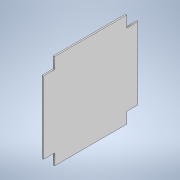
# Autodesk Inventor part: Frame
Saved by Autodesk Inventor 2022 (Build 260153000, 153)
## iProperties
Created: 2022-02-12
Part Number: Frame
Material: Generic
Document SubType Name: Modeling
Designer: ultra
Density: 1 g/cm^3
Appearance: Default
Author: ultra
Autodesk Inventor part; units mm, degrees
ref_plane "YZ Plane" through (0, 0, 0) normal (1, 0, 0) x (0, 1, 0)
ref_plane "XZ Plane" through (0, 0, 0) normal (0, 1, 0) x (-1, 0, 0)
ref_plane "XY Plane" through (0, 0, 0) normal (0, 0, 1) x (1, 0, 0)
sketch "Sketch1" plane through (0, 0, 0) normal (1, 0, 0) x (0, 1, 0)
  line L0 (0, 0) -> (321.6656, 0)
  line L1 (321.6656, 0) -> (321.6656, 321.6656)
  line L2 (321.6656, 321.6656) -> (0, 321.6656)
  line L3 (0, 321.6656) -> (0, 0)
  dimension "d0" = 321.6656
  dimension "d1" = 321.6656
  constraints: 8 end point, 2 parallel, 1 horizontal, 1 perpendicular
  measures "d0" distance of L2.end L1.end
  measures "d1" distance of L1.end L0.end
extrude "Extrusion1" add sketch "Sketch1" along normal blind 4.7752
sketch "Sketch2" plane through (4.7752, 0, 0) normal (1, 0, 0) x (0, 0, -1)
  line L0 (0, 321.6656) -> (-321.6656, 321.6656) projected
  line L1 (-321.6656, 321.6656) -> (-321.6656, 0) projected
  line L2 (-321.6656, 0) -> (0, 0) projected
  line L3 (0, 0) -> (0, 321.6656) projected
  line L4 (-321.6656, 321.6656) -> (-283.5656, 321.6656)
  line L5 (-283.5656, 321.6656) -> (-283.5656, 283.5656)
  line L6 (-283.5656, 283.5656) -> (-321.6656, 283.5656)
  line L7 (-321.6656, 283.5656) -> (-321.6656, 321.6656)
  line L8 (0, 321.6656) -> (-38.1, 321.6656)
  line L9 (-38.1, 321.6656) -> (-38.1, 283.5656)
  line L10 (-38.1, 283.5656) -> (0, 283.5656)
  line L11 (0, 283.5656) -> (0, 321.6656)
  line L12 (0, 0) -> (-38.1, 0)
  line L13 (-38.1, 0) -> (-38.1, 38.1)
  line L14 (-38.1, 38.1) -> (0, 38.1)
  line L15 (0, 38.1) -> (0, 0)
  line L16 (-321.6656, 0) -> (-283.5656, 0)
  line L17 (-283.5656, 0) -> (-283.5656, 38.1)
  line L18 (-283.5656, 38.1) -> (-321.6656, 38.1)
  line L19 (-321.6656, 38.1) -> (-321.6656, 0)
  point P0 (-321.6656, 283.5656)
  point P1 (-38.1, 0)
  point P2 (0, 283.5656)
  dimension "d4" = 38.1
  dimension "d5" = 38.1
  dimension "d6" = 38.1
  dimension "d7" = 38.1
  dimension "d8" = 38.1
  dimension "d9" = 38.1
  dimension "d10" = 38.1
  dimension "d13" = 38.1
  constraints: 32 end point, 8 parallel, 4 horizontal, 4 perpendicular
  measures "d4" distance of L5.end L6.end
  measures "d5" distance of L4.end L5.end
  measures "d6" distance of L10.end L9.end
  measures "d7" distance of L9.end L8.end
  measures "d8" distance of L13.end L14.end
  measures "d9" distance of L12.end L13.end
  measures "d10" distance of L17.end L16.end
  measures "d13" distance of L17.end L18.end
extrude "Extrusion2" cut sketch "Sketch2" against normal blind 4.7752 contours L3 L10 L9 L0 | L5 L6 L1 L0 | L3 L2 L13 L14 | L18 L17 L2 L1
body "Solid1"
